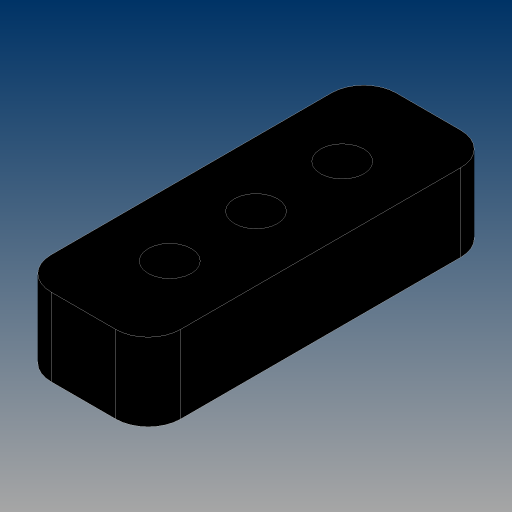
# Autodesk Inventor part: ELEV_026_HARDSTOP1
Saved by Autodesk Inventor 2024.3 (Build 283343000, 343)
## iProperties
Created: 2024-11-29
Part Number: ELEV_026_HARDSTOP1
Material: ABS Plastic
Document SubType Name: Modeling
Designer: Kenji
Density: 1.06 g/cm^3
Appearance: Anodized - Black
Author: Kenji
Autodesk Inventor part; units mm, degrees
ref_plane "YZ Plane" through (0, 0, 0) normal (1, 0, 0) x (0, 1, 0)
ref_plane "XZ Plane" through (0, 0, 0) normal (0, 1, 0) x (-1, 0, 0)
ref_plane "XY Plane" through (0, 0, 0) normal (0, 0, 1) x (1, 0, 0)
sketch "Sketch1" plane through (0, 0, 0) normal (0, 1, 0) x (-1, 0, 0)
  line L0 (4.7625, 0) -> (14.2875, 0)
  line L1 (19.05, -4.7625) -> (19.05, -46.0375)
  line L2 (14.2875, -50.8) -> (4.7625, -50.8)
  line L3 (0, -46.0375) -> (0, -4.7625)
  circle A0 centre (9.525, -12.7) radius 2.54 construction
  circle A1 centre (9.525, -25.4) radius 2.54 construction
  circle A2 centre (9.525, -38.1) radius 2.54 construction
  arc A3 (19.05, -4.7625) -> (14.2875, 0) centre (14.2875, -4.7625) ccw
  arc A4 (14.2875, -50.8) -> (19.05, -46.0375) centre (14.2875, -46.0375) ccw
  arc A5 (0, -46.0375) -> (4.7625, -50.8) centre (4.7625, -46.0375) ccw
  arc A6 (4.7625, 0) -> (0, -4.7625) centre (4.7625, -4.7625) ccw
  point P0 (0, 0)
  point P1 (9.525, -25.4)
  dimension "d0" = 50.8
  dimension "d1" = 19.05
  dimension "d2" = 12.7
  dimension "d3" = 12.7
  dimension "d4" = 12.7
  dimension "d5" = 9.525
  dimension "d6" = 5.08
  dimension "d7" = 4.7625
  constraints: 8 end point, 8 point on circle, 8 tangent, 7 centre point, 5 equal radius, 3 coincident, 2 parallel, 2 point on line, 2 vertical alignment, 1 horizontal, 1 perpendicular
  measures "d0" distance between parallel lines of L2 L0
  measures "d1" distance between parallel lines of L3 L1
  measures "d2" distance of A0.centre A1.centre
  measures "d3" distance of A2.centre A1.centre
  measures "d4" distance from line of L0 A0.centre
  measures "d5" distance from line of L3 A0.centre
  measures "d6" diameter of A0
  measures "d7" radius of A3
extrude "Extrusion1" add sketch "Sketch1" along normal blind 11.43
hole "Hole1" at (-9.525, 0, -38.1) at (-9.525, 0, -25.4) at (-9.525, 0, -38.1) at (-9.525, 0, -12.7) direction (0, 1, 0) diameter 6.35 depth 25.4 counterbore diameter 9.525 counterbore depth 6.35
body "Solid1"
